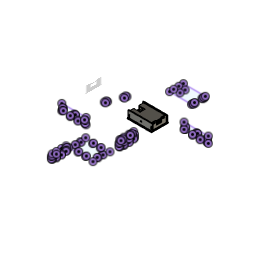
widgetlab1case (Autodesk Fusion 360 design; units mm, degrees)
Autodesk Fusion 360 part; units mm, degrees
(part 1 of 2)
sketch "base" plane through (0, 0, 0) normal (0, 0, 1) x (1, 0, 0)
  line L0 (-26.4, -40.65) -> (26.4, -40.65)
  line L1 (26.4, -40.65) -> (26.4, 40.65)
  line L2 (26.4, 40.65) -> (-26.4, 40.65)
  line L3 (-26.4, 40.65) -> (-26.4, -40.65)
  line L4 (-26.4, -40.65) -> (26.4, -40.65)
  dimension "d5" = 81.3
  dimension "d6" = 52.8
  dimension "d58" = 26.4
  dimension "d59" = 40.65
  dimension "d81" = 52.8
  constraint horizontal L0
  constraint vertical L1
  constraint horizontal L2
  constraint vertical L3
  constraint horizontal L4
  measures "d5" distance of L0.start L2.end
  measures "d6" distance of L1.end L2.end
  measures "d58" distance of origin L1
  measures "d59" distance of origin L2
  measures "d81" distance of L0.start L0.end
extrude "Extrude1" add sketch "base" along normal blind 9.7 makes body 1
sketch "centre groove" plane through (0, 0, 9.7) normal (0, 0, 1) x (1, 0, 0)
  line L0 (-26.4, 40.65) -> (-26.4, -40.65)
  line L1 (-26.4, -40.65) -> (26.4, -40.65)
  line L2 (26.4, -40.65) -> (26.4, 40.65)
  line L3 (26.4, 40.65) -> (-26.4, 40.65)
  line L4 (1.1, -40.65) -> (-1.1, -40.65)
  line L5 (-1.1, -40.65) -> (-1.1, 40.65)
  line L6 (-1.1, 40.65) -> (1.1, 40.65)
  line L7 (1.1, 40.65) -> (1.1, -40.65)
  line L8 (1.1, -40.65) -> (-1.1, 40.65) construction
  line L9 (-1.1, -40.65) -> (1.1, 40.65) construction
  line L10 (-1.1, -40.65) -> (0, -40.65)
  dimension "d9" = 2.2
  dimension "d11" = 1.1
  dimension "d60" = 40.65
  constraint horizontal L4
  constraint perpendicular L4 L5
  constraint parallel L4 L6
  constraint parallel L5 L7
  constraint coincident L8 origin
  constraint coincident L9 origin
  constraint perpendicular L5 L10
  measures "d9" distance of L5.end L6.end
  measures "d11" distance of L4.end L10.end
  measures "d60" distance of L6 origin
extrude "Extrude2" cut sketch "centre groove" against normal blind 3 contours L1 L3 L4 L5 L6 L7 L10 bodies 1
sketch "side dots" plane through (0, 0, 0) normal (0, 0, 1) x (1, 0, 0)
  line L0 (-26.4, 40.65) -> (-26.4, -40.65) construction
  line L1 (26.4, -40.65) -> (26.4, 40.65) construction
  line L2 (26.4, 40.65) -> (1.1, 40.65) construction
  line L3 (-1.1, 40.65) -> (-26.4, 40.65) construction
  line L4 (-1.1, 40.65) -> (1.1, 40.65) construction
  line L5 (-26.4, -40.65) -> (-1.1, -40.65) construction
  line L6 (1.1, -40.65) -> (-1.1, -40.65) construction
  line L7 (1.1, -40.65) -> (26.4, -40.65) construction
  line L8 (-26.4, -40.65) -> (-26.4, -27.3)
  line L9 (-26.4, -27.3) -> (-26.4, 27.3)
  line L10 (0, -40.65) -> (22.3, -40.65)
  line L11 (0, -40.65) -> (-22.3, -40.65)
  line L12 (-26.4, 27.3) -> (-27, 27.3)
  line L13 (-26.4, -27.3) -> (-27, -27.3)
  line L14 (-22.3, -40.65) -> (-22.3, -41.25)
  line L15 (22.3, -40.65) -> (22.3, -41.25)
  circle A0 centre (-27, 27.3) radius 1
  circle A1 centre (-27, -27.3) radius 1
  circle A2 centre (-22.3, -41.25) radius 1
  circle A3 centre (22.3, -41.25) radius 1
  circle A4 centre (0, -41.25) radius 1
  line L16 (0, -40.65) -> (0, -41.25)
  point P0 (-1.1, 40.65)
  point P1 (-1.1, 40.65)
  dimension "d14" = 13.35
  dimension "d15" = 54.6
  dimension "d16" = 22.3
  dimension "d17" = 22.3
  dimension "d18" = 0.6
  dimension "d19" = 0.6
  dimension "d20" = 0.6
  dimension "d21" = 0.6
  dimension "d22" = 2
  dimension "d23" = 2
  dimension "d24" = 2
  dimension "d25" = 2
  dimension "d26" = 2
  dimension "d27" = 0.6
  constraint coincident L0.end L5.start
  constraint perpendicular L5 L8
  constraint parallel L0 L9
  constraint midpoint L6 L10.start
  constraint perpendicular L1 L10
  constraint parallel L5 L11
  constraint perpendicular L9 L12
  constraint perpendicular L0 L13
  constraint perpendicular L11 L14
  constraint perpendicular L10 L15
  constraint coincident L12.end A0.centre
  constraint coincident L13.end A1.centre
  constraint coincident L14.end A2.centre
  constraint coincident L15.end A3.centre
  constraint perpendicular L11 L16
  constraint coincident A4.centre L16.end
  measures "d14" distance of L0.end L8.end
  measures "d15" distance of L8.end L9.end
  measures "d16" distance of L10.start L10.end
  measures "d17" distance of L10.start L11.end
  measures "d18" distance of L9.end L12.end
  measures "d19" distance of L8.end L13.end
  measures "d20" distance of L11.end L14.end
  measures "d21" distance of L10.end L15.end
  measures "d22" diameter of A0
  measures "d23" diameter of A1
  measures "d24" diameter of A2
  measures "d25" diameter of A3
  measures "d26" diameter of A4
  measures "d27" distance of L10.start A4.centre
extrude "Extrude3" add sketch "side dots" along normal blind 4.8 contours L8 L9 A1 | L10 L11 A4 | A0 | A2 | A3 picked at (-27.463, -27.251) picked at (0.0281, -41.7143) bodies 1
sketch "holes" plane through (0, 0, 9.7) normal (0, 0, 1) x (1, 0, 0)
  line L0 (-1.1, -40.65) -> (-1.1, 40.65)
  line L1 (-1.1, 40.65) -> (-26.4, 40.65)
  line L2 (-26.4, 40.65) -> (-26.4, -40.65)
  line L3 (-26.4, -40.65) -> (-1.1, -40.65)
  line L4 (20, 0) -> (2.5, 0)
  line L5 (0, 2.5) -> (0, 20)
  line L6 (0, 0) -> (-26.4, 0) construction
  point P0 (-3.8, 1.27)
  point P1 (-6.34, 1.27)
  point P2 (-8.88, 1.27)
  point P3 (-11.42, 1.27)
  point P4 (-13.96, 1.27)
  point P5 (-3.8, 3.81)
  point P6 (-6.34, 3.81)
  point P7 (-8.88, 3.81)
  point P8 (-11.42, 3.81)
  point P9 (-13.96, 3.81)
  point P10 (-3.8, 6.35)
  point P11 (-6.34, 6.35)
  point P12 (-8.88, 6.35)
  point P13 (-11.42, 6.35)
  point P14 (-13.96, 6.35)
  point P15 (-3.8, 8.89)
  point P16 (-6.34, 8.89)
  point P17 (-8.88, 8.89)
  point P18 (-11.42, 8.89)
  point P19 (-13.96, 8.89)
  point P20 (-3.8, 11.43)
  point P21 (-6.34, 11.43)
  point P22 (-8.88, 11.43)
  point P23 (-11.42, 11.43)
  point P24 (-13.96, 11.43)
  point P25 (-3.8, 13.97)
  point P26 (-6.34, 13.97)
  point P27 (-8.88, 13.97)
  point P28 (-11.42, 13.97)
  point P29 (-13.96, 13.97)
  point P30 (-3.8, 16.51)
  point P31 (-6.34, 16.51)
  point P32 (-8.88, 16.51)
  point P33 (-11.42, 16.51)
  point P34 (-13.96, 16.51)
  point P35 (-3.8, 19.05)
  point P36 (-6.34, 19.05)
  point P37 (-8.88, 19.05)
  point P38 (-11.42, 19.05)
  point P39 (-13.96, 19.05)
  point P40 (-3.8, 21.59)
  point P41 (-6.34, 21.59)
  point P42 (-8.88, 21.59)
  point P43 (-11.42, 21.59)
  point P44 (-13.96, 21.59)
  point P45 (-3.8, 24.13)
  point P46 (-6.34, 24.13)
  point P47 (-8.88, 24.13)
  point P48 (-11.42, 24.13)
  point P49 (-13.96, 24.13)
  point P50 (-3.8, 26.67)
  point P51 (-6.34, 26.67)
  point P52 (-8.88, 26.67)
  point P53 (-11.42, 26.67)
  point P54 (-13.96, 26.67)
  point P55 (-3.8, 29.21)
  point P56 (-6.34, 29.21)
  point P57 (-8.88, 29.21)
  point P58 (-11.42, 29.21)
  point P59 (-13.96, 29.21)
  point P60 (-3.8, 31.75)
  point P61 (-6.34, 31.75)
  point P62 (-8.88, 31.75)
  point P63 (-11.42, 31.75)
  point P64 (-13.96, 31.75)
  point P65 (-3.8, 34.29)
  point P66 (-6.34, 34.29)
  point P67 (-8.88, 34.29)
  point P68 (-11.42, 34.29)
  point P69 (-13.96, 34.29)
  point P70 (-3.8, 36.83)
  point P71 (-6.34, 36.83)
  point P72 (-8.88, 36.83)
  point P73 (-11.42, 36.83)
  point P74 (-13.96, 36.83)
  point P75 (-20.71, 0)
  point P76 (-20.71, -5.08)
  point P77 (-23.25, -5.08)
  point P78 (-20.71, -2.54)
  point P79 (-23.25, -2.54)
  point P80 (-23.25, 0)
  point P81 (-20.71, 2.54)
  point P82 (-23.25, 2.54)
  point P83 (-20.71, 5.08)
  point P84 (-23.25, 5.08)
  point P85 (-23.25, -25.4)
  point P86 (-20.71, -25.4)
  point P87 (-23.25, -27.94)
  point P88 (-20.71, -27.94)
  point P89 (-23.25, -30.48)
  point P90 (-20.71, -30.48)
  point P91 (-23.25, -33.02)
  point P92 (-20.71, -33.02)
  point P93 (-23.25, -35.56)
  point P94 (-20.71, -35.56)
  point P95 (-23.25, -10.16)
  point P96 (-20.71, -10.16)
  point P97 (-23.25, -12.7)
  point P98 (-20.71, -12.7)
  point P99 (-23.25, -15.24)
  point P100 (-20.71, -15.24)
  point P101 (-23.25, -17.78)
  point P102 (-20.71, -17.78)
  point P103 (-23.25, -20.32)
  point P104 (-20.71, -20.32)
  point P105 (-23.25, 20.32)
  point P106 (-20.71, 20.32)
  point P107 (-23.25, 17.78)
  point P108 (-20.71, 17.78)
  point P109 (-23.25, 15.24)
  point P110 (-20.71, 15.24)
  point P111 (-23.25, 12.7)
  point P112 (-20.71, 12.7)
  point P113 (-23.25, 10.16)
  point P114 (-20.71, 10.16)
  point P115 (-23.25, 35.56)
  point P116 (-20.71, 35.56)
  point P117 (-23.25, 33.02)
  point P118 (-20.71, 33.02)
  point P119 (-23.25, 30.48)
  point P120 (-20.71, 30.48)
  point P121 (-23.25, 27.94)
  point P122 (-20.71, 27.94)
  point P123 (-23.25, 25.4)
  point P124 (-20.71, 25.4)
  point P125 (-13.96, -31.75)
  point P126 (-13.96, -34.29)
  point P127 (-13.96, -36.83)
  point P128 (-3.8, -31.75)
  point P129 (-11.42, -31.75)
  point P130 (-3.8, -24.13)
  point P131 (-3.8, -36.83)
  point P132 (-6.34, -21.59)
  point P133 (-3.8, -29.21)
  point P134 (-8.88, -29.21)
  point P135 (-6.34, -36.83)
  point P136 (-8.88, -31.75)
  point P137 (-13.96, -21.59)
  point P138 (-13.96, -3.81)
  point P139 (-8.88, -21.59)
  point P140 (-3.8, -34.29)
  point P141 (-8.88, -34.29)
  point P142 (-11.42, -36.83)
  point P143 (-11.42, -8.89)
  point P144 (-8.88, -11.43)
  point P145 (-8.88, -36.83)
  point P146 (-13.96, -6.35)
  point P147 (-13.96, -11.43)
  point P148 (-6.34, -24.13)
  point P149 (-6.34, -29.21)
  point P150 (-13.96, -1.27)
  point P151 (-8.88, -26.67)
  point P152 (-3.8, -21.59)
  point P153 (-11.42, -34.29)
  point P154 (-6.34, -26.67)
  point P155 (-11.42, -13.97)
  point P156 (-6.34, -31.75)
  point P157 (-13.96, -16.51)
  point P158 (-11.42, -11.43)
  point P159 (-11.42, -26.67)
  point P160 (-6.34, -19.05)
  point P161 (-8.88, -19.05)
  point P162 (-13.96, -8.89)
  point P163 (-11.42, -19.05)
  point P164 (-11.42, -24.13)
  point P165 (-11.42, -21.59)
  point P166 (-13.96, -26.67)
  point P167 (-13.96, -29.21)
  point P168 (-3.8, -26.67)
  point P169 (-11.42, -1.27)
  point P170 (-8.88, -8.89)
  point P171 (-11.42, -29.21)
  point P172 (-11.42, -6.35)
  point P173 (-6.34, -34.29)
  point P174 (-13.96, -24.13)
  point P175 (-13.96, -13.97)
  point P176 (-8.88, -1.27)
  point P177 (-3.8, -8.89)
  point P178 (-3.8, -6.35)
  point P179 (-8.88, -6.35)
  point P180 (-11.42, -3.81)
  point P181 (-8.88, -16.51)
  point P182 (-6.34, -1.27)
  point P183 (-11.42, -16.51)
  point P184 (-3.8, -3.81)
  point P185 (-6.34, -8.89)
  point P186 (-6.34, -6.35)
  point P187 (-3.8, -11.43)
  point P188 (-6.34, -11.43)
  point P189 (-6.34, -16.51)
  point P190 (-8.88, -3.81)
  point P191 (-8.88, -24.13)
  point P192 (-6.34, -13.97)
  point P193 (-8.88, -13.97)
  point P194 (-3.8, -19.05)
  point P195 (-3.8, -16.51)
  point P196 (-3.8, -13.97)
  point P197 (-6.34, -3.81)
  point P198 (-13.96, -19.05)
  point P199 (-3.8, -1.27)
  point P200 (3.8, -21.59)
  point P201 (8.88, 34.29)
  point P202 (13.96, 1.27)
  point P203 (20.71, -15.24)
  point P204 (23.25, 5.08)
  point P205 (6.34, 13.97)
  point P206 (11.42, -36.83)
  point P207 (3.8, -6.35)
  point P208 (3.8, 1.27)
  point P209 (23.25, -27.94)
  point P210 (3.8, 36.83)
  point P211 (11.42, -29.21)
  point P212 (6.34, 3.81)
  point P213 (11.42, -8.89)
  point P214 (13.96, -13.97)
  point P215 (23.25, 17.78)
  point P216 (8.88, 29.21)
  point P217 (20.71, 10.16)
  point P218 (13.96, 36.83)
  point P219 (3.8, -26.67)
  point P220 (8.88, -24.13)
  point P221 (23.25, -17.78)
  point P222 (13.96, -31.75)
  point P223 (8.88, 8.89)
  point P224 (3.8, 31.75)
  point P225 (8.88, 31.75)
  point P226 (20.71, -12.7)
  point P227 (6.34, -16.51)
  point P228 (11.42, -13.97)
  point P229 (11.42, -16.51)
  point P230 (3.8, -3.81)
  point P231 (20.71, 17.78)
  point P232 (6.34, -11.43)
  point P233 (3.8, 24.13)
  point P234 (13.96, -34.29)
  point P235 (23.25, -20.32)
  point P236 (20.71, -30.48)
  point P237 (6.34, 29.21)
  point P238 (20.71, 33.02)
  point P239 (6.34, 11.43)
  point P240 (8.88, 16.51)
  point P241 (13.96, 26.67)
  point P242 (11.42, 6.35)
  point P243 (8.88, -8.89)
  point P244 (11.42, -11.43)
  point P245 (13.96, -21.59)
  point P246 (13.96, 34.29)
  point P247 (3.8, -31.75)
  point P248 (11.42, -31.75)
  point P249 (6.34, -21.59)
  point P250 (11.42, 1.27)
  point P251 (20.71, -20.32)
  point P252 (8.88, -26.67)
  point P253 (6.34, -34.29)
  point P254 (3.8, 8.89)
  point P255 (13.96, -19.05)
  point P256 (23.25, -25.4)
  point P257 (6.34, -29.21)
  point P258 (23.25, -33.02)
  point P259 (3.8, 34.29)
  point P260 (8.88, -11.43)
  point P261 (23.25, 35.56)
  point P262 (3.8, -1.27)
  point P263 (13.96, 29.21)
  point P264 (3.8, 29.21)
  point P265 (3.8, -34.29)
  point P266 (8.88, -29.21)
  point P267 (23.25, 33.02)
  point P268 (13.96, -24.13)
  point P269 (11.42, 36.83)
  point P270 (8.88, -13.97)
  point P271 (8.88, -31.75)
  point P272 (13.96, -26.67)
  point P273 (6.34, -26.67)
  point P274 (3.8, 19.05)
  point P275 (3.8, 6.35)
  point P276 (11.42, -24.13)
  point P277 (20.71, -27.94)
  point P278 (8.88, 24.13)
  point P279 (6.34, 1.27)
  point P280 (6.34, -36.83)
  point P281 (11.42, 34.29)
  point P282 (8.88, 3.81)
  point P283 (23.25, -30.48)
  point P284 (11.42, -34.29)
  point P285 (3.8, -8.89)
  point P286 (6.34, -1.27)
  point P287 (8.88, -3.81)
  point P288 (3.8, 16.51)
  point P289 (11.42, 29.21)
  point P290 (8.88, 11.43)
  point P291 (23.25, 30.48)
  point P292 (3.8, -11.43)
  point P293 (20.71, -35.56)
  point P294 (13.96, -16.51)
  point P295 (23.25, -35.56)
  point P296 (3.8, -24.13)
  point P297 (13.96, -11.43)
  point P298 (3.8, 11.43)
  point P299 (20.71, 35.56)
  point P300 (13.96, -36.83)
  point P301 (6.34, -6.35)
  point P302 (3.8, -36.83)
  point P303 (11.42, 31.75)
  point P304 (6.34, -8.89)
  point P305 (3.8, -16.51)
  point P306 (13.96, 21.59)
  point P307 (11.42, -26.67)
  point P308 (6.34, -31.75)
  point P309 (8.88, -1.27)
  point P310 (8.88, 36.83)
  point P311 (11.42, -21.59)
  point P312 (20.71, -25.4)
  point P313 (11.42, -6.35)
  point P314 (20.71, 5.08)
  point P315 (11.42, 21.59)
  point P316 (13.96, 16.51)
  point P317 (13.96, 6.35)
  point P318 (11.42, 11.43)
  point P319 (8.88, 19.05)
  point P320 (6.34, 24.13)
  point P321 (13.96, -1.27)
  point P322 (23.25, 2.54)
  point P323 (23.25, -2.54)
  point P324 (11.42, 16.51)
  point P325 (11.42, 8.89)
  point P326 (13.96, 3.81)
  point P327 (13.96, 19.05)
  point P328 (20.71, -2.54)
  point P329 (13.96, 11.43)
  point P330 (13.96, -3.81)
  point P331 (23.25, 10.16)
  point P332 (20.71, 15.24)
  point P333 (23.25, 0)
  point P334 (13.96, 13.97)
  point P335 (11.42, -3.81)
  point P336 (11.42, -1.27)
  point P337 (11.42, 19.05)
  point P338 (20.71, -17.78)
  point P339 (23.25, 20.32)
  point P340 (23.25, 15.24)
  point P341 (8.88, 26.67)
  point P342 (6.34, 19.05)
  point P343 (6.34, 21.59)
  point P344 (20.71, 25.4)
  point P345 (13.96, 8.89)
  point P346 (20.71, -10.16)
  point P347 (23.25, -5.08)
  point P348 (11.42, 26.67)
  point P349 (20.71, 2.54)
  point P350 (6.34, 26.67)
  point P351 (20.71, 20.32)
  point P352 (11.42, -19.05)
  point P353 (11.42, 13.97)
  point P354 (23.25, -12.7)
  point P355 (13.96, 24.13)
  point P356 (8.88, 21.59)
  point P357 (20.71, 0)
  point P358 (13.96, -6.35)
  point P359 (20.71, 12.7)
  point P360 (23.25, 25.4)
  point P361 (20.71, -5.08)
  point P362 (23.25, 12.7)
  point P363 (3.8, 21.59)
  point P364 (11.42, 3.81)
  point P365 (3.8, 26.67)
  point P366 (8.88, -16.51)
  point P367 (3.8, 13.97)
  point P368 (6.34, 16.51)
  point P369 (23.25, -15.24)
  point P370 (6.34, 31.75)
  point P371 (6.34, 34.29)
  point P372 (13.96, -29.21)
  point P373 (6.34, -19.05)
  point P374 (20.71, -33.02)
  point P375 (3.8, -19.05)
  point P376 (8.88, 6.35)
  point P377 (13.96, 31.75)
  point P378 (20.71, 30.48)
  point P379 (8.88, -6.35)
  point P380 (3.8, 3.81)
  point P381 (8.88, -34.29)
  point P382 (8.88, 1.27)
  point P383 (6.34, -3.81)
  point P384 (6.34, -13.97)
  point P385 (8.88, -19.05)
  point P386 (8.88, 13.97)
  point P387 (6.34, 6.35)
  point P388 (20.71, 27.94)
  point P389 (23.25, -10.16)
  point P390 (23.25, 27.94)
  point P391 (6.34, -24.13)
  point P392 (8.88, -21.59)
  point P393 (13.96, -8.89)
  point P394 (11.42, 24.13)
  point P395 (8.88, -36.83)
  point P396 (6.34, 36.83)
  point P397 (6.34, 8.89)
  point P398 (3.8, -13.97)
  point P399 (3.8, -29.21)
  dimension "d32" = 3.8
  dimension "d33" = 1.27
  dimension "d36" = -10.16
  dimension "d37" = 35.56
  dimension "d39" = 6.75
  dimension "d42" = -2.54
  dimension "d43" = 5.08
  dimension "d46" = 0
  dimension "d47" = 30.48
  constraint symmetric P0 L4 P199
  constraint symmetric P1 L4 P182
  constraint symmetric P2 L4 P176
  constraint symmetric P3 L4 P169
  constraint symmetric P4 L4 P150
  constraint symmetric P5 L4 P184
  constraint symmetric P6 L4 P197
  constraint symmetric P7 L4 P190
  constraint symmetric P8 L4 P180
  constraint symmetric P9 L4 P138
  constraint symmetric P10 L4 P178
  constraint symmetric P11 L4 P186
  constraint symmetric P12 L4 P179
  constraint symmetric P13 L4 P172
  constraint symmetric P14 L4 P146
  constraint symmetric P15 L4 P177
  constraint symmetric P16 L4 P185
  constraint symmetric P17 L4 P170
  constraint symmetric P18 L4 P143
  constraint symmetric P19 L4 P162
  constraint symmetric P20 L4 P187
  constraint symmetric P21 L4 P188
  constraint symmetric P22 L4 P144
  constraint symmetric P23 L4 P158
  constraint symmetric P24 L4 P147
  constraint symmetric P25 L4 P196
  constraint symmetric P26 L4 P192
  constraint symmetric P27 L4 P193
  constraint symmetric P28 L4 P155
  constraint symmetric P29 L4 P175
  constraint symmetric P30 L4 P195
  constraint symmetric P31 L4 P189
  constraint symmetric P32 L4 P181
  constraint symmetric P33 L4 P183
  constraint symmetric P34 L4 P157
  constraint symmetric P35 L4 P194
  constraint symmetric P36 L4 P160
  constraint symmetric P37 L4 P161
  constraint symmetric P38 L4 P163
  constraint symmetric P39 L4 P198
  constraint symmetric P40 L4 P152
  constraint symmetric P41 L4 P132
  constraint symmetric P42 L4 P139
  constraint symmetric P43 L4 P165
  constraint symmetric P44 L4 P137
  constraint symmetric P45 L4 P130
  constraint symmetric P46 L4 P148
  constraint symmetric P47 L4 P191
  constraint symmetric P48 L4 P164
  constraint symmetric P49 L4 P174
  constraint symmetric P50 L4 P168
  constraint symmetric P51 L4 P154
  constraint symmetric P52 L4 P151
  constraint symmetric P53 L4 P159
  constraint symmetric P54 L4 P166
  constraint symmetric P55 L4 P133
  constraint symmetric P56 L4 P149
  constraint symmetric P57 L4 P134
  constraint symmetric P58 L4 P171
  constraint symmetric P59 L4 P167
  constraint symmetric P60 L4 P128
  constraint symmetric P61 L4 P156
  constraint symmetric P62 L4 P136
  constraint symmetric P63 L4 P129
  constraint symmetric P64 L4 P125
  constraint symmetric P65 L4 P140
  constraint symmetric P66 L4 P173
  constraint symmetric P67 L4 P141
  constraint symmetric P68 L4 P153
  constraint symmetric P69 L4 P126
  constraint symmetric P70 L4 P131
  constraint symmetric P71 L4 P135
  constraint symmetric P72 L4 P145
  constraint symmetric P73 L4 P142
  constraint symmetric P74 L4 P127
  constraint symmetric P0 L5 P208
  constraint symmetric P1 L5 P279
  constraint symmetric P2 L5 P382
  constraint symmetric P3 L5 P250
  constraint symmetric P4 L5 P202
  constraint symmetric P5 L5 P380
  constraint symmetric P6 L5 P212
  constraint symmetric P7 L5 P282
  constraint symmetric P8 L5 P364
  constraint symmetric P9 L5 P326
  constraint symmetric P10 L5 P275
  constraint symmetric P11 L5 P387
  constraint symmetric P12 L5 P376
  constraint symmetric P13 L5 P242
  constraint symmetric P14 L5 P317
  constraint symmetric P15 L5 P254
  constraint symmetric P16 L5 P397
  constraint symmetric P17 L5 P223
  constraint symmetric P18 L5 P325
  constraint symmetric P19 L5 P345
  constraint symmetric P20 L5 P298
  constraint symmetric P21 L5 P239
  constraint symmetric P22 L5 P290
  constraint symmetric P23 L5 P318
  constraint symmetric P24 L5 P329
  constraint symmetric P25 L5 P367
  constraint symmetric P26 L5 P205
  constraint symmetric P27 L5 P386
  constraint symmetric P28 L5 P353
  constraint symmetric P29 L5 P334
  constraint symmetric P30 L5 P288
  constraint symmetric P31 L5 P368
  constraint symmetric P32 L5 P240
  constraint symmetric P33 L5 P324
  constraint symmetric P34 L5 P316
  constraint symmetric P35 L5 P274
  constraint symmetric P36 L5 P342
  constraint symmetric P37 L5 P319
  constraint symmetric P38 L5 P337
  constraint symmetric P39 L5 P327
  constraint symmetric P40 L5 P363
  constraint symmetric P41 L5 P343
  constraint symmetric P42 L5 P356
  constraint symmetric P43 L5 P315
  constraint symmetric P44 L5 P306
  constraint symmetric P45 L5 P233
  constraint symmetric P46 L5 P320
  constraint symmetric P47 L5 P278
  constraint symmetric P48 L5 P394
  constraint symmetric P49 L5 P355
  constraint symmetric P50 L5 P365
  constraint symmetric P51 L5 P350
  constraint symmetric P52 L5 P341
  constraint symmetric P53 L5 P348
  constraint symmetric P54 L5 P241
  constraint symmetric P55 L5 P264
  constraint symmetric P56 L5 P237
  constraint symmetric P57 L5 P216
  constraint symmetric P58 L5 P289
  constraint symmetric P59 L5 P263
  constraint symmetric P60 L5 P224
  constraint symmetric P61 L5 P370
  constraint symmetric P62 L5 P225
  constraint symmetric P63 L5 P303
  constraint symmetric P64 L5 P377
  constraint symmetric P65 L5 P259
  constraint symmetric P66 L5 P371
  constraint symmetric P67 L5 P201
  constraint symmetric P68 L5 P281
  constraint symmetric P69 L5 P246
  constraint symmetric P70 L5 P210
  constraint symmetric P71 L5 P396
  constraint symmetric P72 L5 P310
  constraint symmetric P73 L5 P269
  constraint symmetric P74 L5 P218
  constraint symmetric P75 L5 P357
  constraint symmetric P76 L5 P361
  constraint symmetric P77 L5 P347
  constraint symmetric P78 L5 P328
  constraint symmetric P79 L5 P323
  constraint symmetric P80 L5 P333
  constraint symmetric P81 L5 P349
  constraint symmetric P82 L5 P322
  constraint symmetric P83 L5 P314
  constraint symmetric P84 L5 P204
  constraint symmetric P85 L5 P256
  constraint symmetric P86 L5 P312
  constraint symmetric P87 L5 P209
  constraint symmetric P88 L5 P277
  constraint symmetric P89 L5 P283
  constraint symmetric P90 L5 P236
  constraint symmetric P91 L5 P258
  constraint symmetric P92 L5 P374
  constraint symmetric P93 L5 P295
  constraint symmetric P94 L5 P293
  constraint symmetric P95 L5 P389
  constraint symmetric P96 L5 P346
  constraint symmetric P97 L5 P354
  constraint symmetric P98 L5 P226
  constraint symmetric P99 L5 P369
  constraint symmetric P100 L5 P203
  constraint symmetric P101 L5 P221
  constraint symmetric P102 L5 P338
  constraint symmetric P103 L5 P235
  constraint symmetric P104 L5 P251
  constraint symmetric P105 L5 P339
  constraint symmetric P106 L5 P351
  constraint symmetric P107 L5 P215
  constraint symmetric P108 L5 P231
  constraint symmetric P109 L5 P340
  constraint symmetric P110 L5 P332
  constraint symmetric P111 L5 P362
  constraint symmetric P112 L5 P359
  constraint symmetric P113 L5 P331
  constraint symmetric P114 L5 P217
  constraint symmetric P115 L5 P261
  constraint symmetric P116 L5 P299
  constraint symmetric P117 L5 P267
  constraint symmetric P118 L5 P238
  constraint symmetric P119 L5 P291
  constraint symmetric P120 L5 P378
  constraint symmetric P121 L5 P390
  constraint symmetric P122 L5 P388
  constraint symmetric P123 L5 P360
  constraint symmetric P124 L5 P344
  constraint symmetric P125 L5 P222
  constraint symmetric P126 L5 P234
  constraint symmetric P127 L5 P300
  constraint symmetric P128 L5 P247
  constraint symmetric P129 L5 P248
  constraint symmetric P130 L5 P296
  constraint symmetric P131 L5 P302
  constraint symmetric P132 L5 P249
  constraint symmetric P133 L5 P399
  constraint symmetric P134 L5 P266
  constraint symmetric P135 L5 P280
  constraint symmetric P136 L5 P271
  constraint symmetric P137 L5 P245
  constraint symmetric P138 L5 P330
  constraint symmetric P139 L5 P392
  constraint symmetric P140 L5 P265
  constraint symmetric P141 L5 P381
  constraint symmetric P142 L5 P206
  constraint symmetric P143 L5 P213
  constraint symmetric P144 L5 P260
  constraint symmetric P145 L5 P395
  constraint symmetric P146 L5 P358
  constraint symmetric P147 L5 P297
  constraint symmetric P148 L5 P391
  constraint symmetric P149 L5 P257
  constraint symmetric P150 L5 P321
  constraint symmetric P151 L5 P252
  constraint symmetric P152 L5 P200
  constraint symmetric P153 L5 P284
  constraint symmetric P154 L5 P273
  constraint symmetric P155 L5 P228
  constraint symmetric P156 L5 P308
  constraint symmetric P157 L5 P294
  constraint symmetric P158 L5 P244
  constraint symmetric P159 L5 P307
  constraint symmetric P160 L5 P373
  constraint symmetric P161 L5 P385
  constraint symmetric P162 L5 P393
  constraint symmetric P163 L5 P352
  constraint symmetric P164 L5 P276
  constraint symmetric P165 L5 P311
  constraint symmetric P166 L5 P272
  constraint symmetric P167 L5 P372
  constraint symmetric P168 L5 P219
  constraint symmetric P169 L5 P336
  constraint symmetric P170 L5 P243
  constraint symmetric P171 L5 P211
  constraint symmetric P172 L5 P313
  constraint symmetric P173 L5 P253
  constraint symmetric P174 L5 P268
  constraint symmetric P175 L5 P214
  constraint symmetric P176 L5 P309
  constraint symmetric P177 L5 P285
  constraint symmetric P178 L5 P207
  constraint symmetric P179 L5 P379
  constraint symmetric P180 L5 P335
  constraint symmetric P181 L5 P366
  constraint symmetric P182 L5 P286
  constraint symmetric P183 L5 P229
  constraint symmetric P184 L5 P230
  constraint symmetric P185 L5 P304
  constraint symmetric P186 L5 P301
  constraint symmetric P187 L5 P292
  constraint symmetric P188 L5 P232
  constraint symmetric P189 L5 P227
  constraint symmetric P190 L5 P287
  constraint symmetric P191 L5 P220
  constraint symmetric P192 L5 P384
  constraint symmetric P193 L5 P270
  constraint symmetric P194 L5 P375
  constraint symmetric P195 L5 P305
  constraint symmetric P196 L5 P398
  constraint symmetric P197 L5 P383
  constraint symmetric P198 L5 P255
  constraint symmetric P199 L5 P262
  constraint coincident L6.start origin
  constraint midpoint L2 L6.end
  constraint coincident P80 L6
  measures "d24" diameter of P81
  measures "d25" diameter of P313
  measures "d32" horizontal distance of L6.start P0
  measures "d33" vertical distance of L6.start P0
  measures "d39" horizontal distance of P4 P75
hole "Hole1" at (-6.34, -1.27, 9.7) at (-20.71, -10.16, 9.7) at (-3.8, 13.97, 9.7) at (-13.96, 8.89, 9.7) at (-6.34, -13.97, 9.7) at (-8.88, -24.13, 9.7) at (-3.8, -3.81, 9.7) at (-13.96, 34.29, 9.7) at (-23.25, -35.56, 9.7) at (-20.71, -33.02, 9.7) at (-20.71, -12.7, 9.7) at (-3.8, 11.43, 9.7) at (-20.71, 20.32, 9.7) at (-8.88, -1.27, 9.7) at (-13.96, 13.97, 9.7) at (-11.42, 13.97, 9.7) at (-8.88, 36.83, 9.7) at (-3.8, -36.83, 9.7) at (-8.88, 11.43, 9.7) at (-20.71, -30.48, 9.7) at (-13.96, 29.21, 9.7) at (-13.96, -13.97, 9.7) at (-3.8, -21.59, 9.7) at (-13.96, -1.27, 9.7) at (-6.34, -16.51, 9.7) at (-3.8, 3.81, 9.7) at (-11.42, 19.05, 9.7) at (-23.25, -17.78, 9.7) at (-3.8, -31.75, 9.7) at (-11.42, -24.13, 9.7) at (-8.88, 6.35, 9.7) at (-6.34, -6.35, 9.7) at (-3.8, 34.29, 9.7) at (-13.96, -11.43, 9.7) at (-13.96, 19.05, 9.7) at (-8.88, -11.43, 9.7) at (-3.8, -24.13, 9.7) at (-8.88, -3.81, 9.7) at (-13.96, -21.59, 9.7) at (-13.96, 36.83, 9.7) at (-6.34, 8.89, 9.7) at (-8.88, -13.97, 9.7) at (-20.71, -35.56, 9.7) at (-3.8, 16.51, 9.7) at (-8.88, 29.21, 9.7) at (-6.34, -31.75, 9.7) at (-20.71, 12.7, 9.7) at (-23.25, -25.4, 9.7) at (-6.34, -24.13, 9.7) at (-20.71, -20.32, 9.7) at (-23.25, 20.32, 9.7) at (-8.88, -16.51, 9.7) at (-11.42, -36.83, 9.7) at (-6.34, -36.83, 9.7) at (-3.8, -19.05, 9.7) at (-3.8, 19.05, 9.7) at (-8.88, -6.35, 9.7) at (-20.71, -25.4, 9.7) at (-6.34, 29.21, 9.7) at (-11.42, -16.51, 9.7) at (-3.8, 1.27, 9.7) at (-6.34, -21.59, 9.7) at (-6.34, -11.43, 9.7) at (-8.88, -31.75, 9.7) at (-6.34, 6.35, 9.7) at (-6.34, 24.13, 9.7) at (-13.96, -29.21, 9.7) at (-8.88, 26.67, 9.7) at (-13.96, 31.75, 9.7) at (-13.96, 21.59, 9.7) at (-20.71, 10.16, 9.7) at (-3.8, 29.21, 9.7) at (-11.42, 26.67, 9.7) at (-20.71, -27.94, 9.7) at (-6.34, -26.67, 9.7) at (-3.8, 26.67, 9.7) at (-3.8, 6.35, 9.7) at (-8.88, 3.81, 9.7) at (-8.88, -34.29, 9.7) at (-23.25, -5.08, 9.7) at (-3.8, -1.27, 9.7) at (-13.96, -8.89, 9.7) at (-8.88, -21.59, 9.7) at (-11.42, -21.59, 9.7) at (-3.8, 24.13, 9.7) at (-11.42, 8.89, 9.7) at (-6.34, 3.81, 9.7) at (-8.88, 31.75, 9.7) at (-6.34, 31.75, 9.7) at (-20.71, 30.48, 9.7) at (-13.96, 26.67, 9.7) at (-13.96, 6.35, 9.7) at (-11.42, 16.51, 9.7) at (-23.25, 10.16, 9.7) at (-13.96, 16.51, 9.7) at (-11.42, 31.75, 9.7) at (-11.42, 29.21, 9.7) at (-23.25, 5.08, 9.7) at (-13.96, -19.05, 9.7) at (-11.42, -11.43, 9.7) at (-11.42, -26.67, 9.7) at (-20.71, -15.24, 9.7) at (-23.25, 27.94, 9.7) at (-6.34, 19.05, 9.7) at (-13.96, -3.81, 9.7) at (-23.25, 33.02, 9.7) at (-11.42, 21.59, 9.7) at (-11.42, -3.81, 9.7) at (-23.25, 35.56, 9.7) at (-6.34, 34.29, 9.7) at (-13.96, 1.27, 9.7) at (-13.96, 24.13, 9.7) at (-11.42, -6.35, 9.7) at (-13.96, 3.81, 9.7) at (-23.25, 2.54, 9.7) at (-13.96, 11.43, 9.7) at (-20.71, 2.54, 9.7) at (-13.96, -6.35, 9.7) at (-23.25, 15.24, 9.7) at (-11.42, 6.35, 9.7) at (-20.71, 15.24, 9.7) at (-11.42, 11.43, 9.7) at (-23.25, 0, 9.7) at (-20.71, 0, 9.7) at (-20.71, -5.08, 9.7) at (-11.42, -1.27, 9.7) at (-8.88, 16.51, 9.7) at (-20.71, 33.02, 9.7) at (-8.88, 21.59, 9.7) at (-23.25, -33.02, 9.7) at (-13.96, -24.13, 9.7) at (-20.71, -17.78, 9.7) at (-13.96, -34.29, 9.7) at (-11.42, 1.27, 9.7) at (-13.96, -31.75, 9.7) at (-23.25, 25.4, 9.7) at (-11.42, 36.83, 9.7) at (-8.88, -8.89, 9.7) at (-3.8, -26.67, 9.7) at (-3.8, -16.51, 9.7) at (-23.25, -20.32, 9.7) at (-3.8, -29.21, 9.7) at (-6.34, -34.29, 9.7) at (-20.71, 5.08, 9.7) at (-6.34, 1.27, 9.7) at (-11.42, 34.29, 9.7) at (-8.88, 24.13, 9.7) at (-3.8, 21.59, 9.7) at (-3.8, -6.35, 9.7) at (-11.42, -31.75, 9.7) at (-11.42, -13.97, 9.7) at (-11.42, 3.81, 9.7) at (-13.96, -16.51, 9.7) at (-13.96, -26.67, 9.7) at (-6.34, 16.51, 9.7) at (-6.34, 13.97, 9.7) at (-23.25, -2.54, 9.7) at (-3.8, 8.89, 9.7) at (-11.42, -29.21, 9.7) at (-8.88, 34.29, 9.7) at (-8.88, 1.27, 9.7) at (-23.25, -30.48, 9.7) at (-11.42, -19.05, 9.7) at (-20.71, 27.94, 9.7) at (-8.88, -36.83, 9.7) at (-3.8, 31.75, 9.7) at (-20.71, 35.56, 9.7) at (-6.34, -8.89, 9.7) at (-11.42, -34.29, 9.7) at (-20.71, -2.54, 9.7) at (-6.34, -3.81, 9.7) at (-8.88, -29.21, 9.7) at (-20.71, 25.4, 9.7) at (-6.34, 11.43, 9.7) at (-23.25, -12.7, 9.7) at (-6.34, 26.67, 9.7) at (-3.8, -13.97, 9.7) at (-6.34, -19.05, 9.7) at (-6.34, -29.21, 9.7) at (-3.8, -11.43, 9.7) at (-23.25, 30.48, 9.7) at (-23.25, -10.16, 9.7) at (-23.25, 12.7, 9.7) at (-20.71, 17.78, 9.7) at (-23.25, 17.78, 9.7) at (-11.42, -8.89, 9.7) at (-6.34, 21.59, 9.7) at (-8.88, 19.05, 9.7) at (-13.96, -36.83, 9.7) at (-11.42, 24.13, 9.7) at (-23.25, -15.24, 9.7) at (-23.25, -27.94, 9.7) at (-3.8, -34.29, 9.7) at (-3.8, 36.83, 9.7) at (-3.8, -8.89, 9.7) at (-8.88, -26.67, 9.7) at (-8.88, 8.89, 9.7) at (-8.88, -19.05, 9.7) at (-6.34, 36.83, 9.7) at (-8.88, 13.97, 9.7) direction (0, 0, -1) diameter 1.524 depth 7 tip angle 180 bodies 1
hole "Hole2" at (6.34, -11.43, 9.7) at (20.71, 15.24, 9.7) at (23.25, 2.54, 9.7) at (23.25, 0, 9.7) at (6.34, 34.29, 9.7) at (6.34, -26.67, 9.7) at (8.88, 11.43, 9.7) at (3.8, 1.27, 9.7) at (8.88, 26.67, 9.7) at (23.25, -17.78, 9.7) at (20.71, -33.02, 9.7) at (6.34, 13.97, 9.7) at (3.8, -8.89, 9.7) at (8.88, -26.67, 9.7) at (23.25, 17.78, 9.7) at (20.71, 17.78, 9.7) at (8.88, -29.21, 9.7) at (13.96, -21.59, 9.7) at (3.8, -29.21, 9.7) at (3.8, 16.51, 9.7) at (8.88, -31.75, 9.7) at (3.8, 26.67, 9.7) at (3.8, -16.51, 9.7) at (6.34, 8.89, 9.7) at (6.34, -6.35, 9.7) at (11.42, 1.27, 9.7) at (23.25, 25.4, 9.7) at (8.88, -1.27, 9.7) at (13.96, 6.35, 9.7) at (8.88, 3.81, 9.7) at (6.34, -16.51, 9.7) at (13.96, -3.81, 9.7) at (8.88, -8.89, 9.7) at (23.25, -10.16, 9.7) at (3.8, -26.67, 9.7) at (6.34, -1.27, 9.7) at (11.42, -6.35, 9.7) at (6.34, 6.35, 9.7) at (11.42, -8.89, 9.7) at (6.34, -21.59, 9.7) at (13.96, 1.27, 9.7) at (6.34, 26.67, 9.7) at (3.8, 3.81, 9.7) at (23.25, 12.7, 9.7) at (11.42, -31.75, 9.7) at (13.96, -19.05, 9.7) at (13.96, 26.67, 9.7) at (11.42, -13.97, 9.7) at (13.96, -24.13, 9.7) at (11.42, 13.97, 9.7) at (11.42, 11.43, 9.7) at (13.96, 24.13, 9.7) at (23.25, -15.24, 9.7) at (8.88, 6.35, 9.7) at (20.71, 12.7, 9.7) at (20.71, -20.32, 9.7) at (20.71, 33.02, 9.7) at (11.42, 34.29, 9.7) at (20.71, 10.16, 9.7) at (8.88, -13.97, 9.7) at (11.42, 19.05, 9.7) at (23.25, -30.48, 9.7) at (3.8, 29.21, 9.7) at (20.71, -12.7, 9.7) at (13.96, 34.29, 9.7) at (11.42, 31.75, 9.7) at (6.34, 31.75, 9.7) at (11.42, -34.29, 9.7) at (23.25, 20.32, 9.7) at (13.96, -36.83, 9.7) at (11.42, -11.43, 9.7) at (13.96, -26.67, 9.7) at (13.96, -31.75, 9.7) at (6.34, -29.21, 9.7) at (8.88, -6.35, 9.7) at (13.96, 16.51, 9.7) at (13.96, 36.83, 9.7) at (23.25, 30.48, 9.7) at (13.96, 19.05, 9.7) at (6.34, 3.81, 9.7) at (6.34, 19.05, 9.7) at (13.96, 31.75, 9.7) at (13.96, -6.35, 9.7) at (11.42, -29.21, 9.7) at (13.96, -13.97, 9.7) at (3.8, -21.59, 9.7) at (20.71, -27.94, 9.7) at (3.8, 36.83, 9.7) at (3.8, 24.13, 9.7) at (8.88, 36.83, 9.7) at (6.34, 36.83, 9.7) at (11.42, -24.13, 9.7) at (11.42, -36.83, 9.7) at (20.71, -15.24, 9.7) at (3.8, 31.75, 9.7) at (8.88, 21.59, 9.7) at (8.88, -36.83, 9.7) at (20.71, -35.56, 9.7) at (23.25, -25.4, 9.7) at (8.88, 24.13, 9.7) at (20.71, 27.94, 9.7) at (13.96, -34.29, 9.7) at (23.25, -35.56, 9.7) at (20.71, 30.48, 9.7) at (11.42, 26.67, 9.7) at (23.25, -20.32, 9.7) at (6.34, -24.13, 9.7) at (11.42, -16.51, 9.7) at (3.8, 8.89, 9.7) at (20.71, 25.4, 9.7) at (3.8, -11.43, 9.7) at (8.88, -11.43, 9.7) at (23.25, -33.02, 9.7) at (20.71, 2.54, 9.7) at (3.8, 6.35, 9.7) at (3.8, -36.83, 9.7) at (3.8, -6.35, 9.7) at (11.42, 3.81, 9.7) at (3.8, -24.13, 9.7) at (8.88, 13.97, 9.7) at (20.71, -2.54, 9.7) at (13.96, 11.43, 9.7) at (6.34, 11.43, 9.7) at (8.88, 34.29, 9.7) at (20.71, -30.48, 9.7) at (3.8, -3.81, 9.7) at (23.25, 33.02, 9.7) at (8.88, 19.05, 9.7) at (11.42, -19.05, 9.7) at (3.8, -34.29, 9.7) at (11.42, 21.59, 9.7) at (6.34, 24.13, 9.7) at (8.88, 29.21, 9.7) at (13.96, -16.51, 9.7) at (20.71, 0, 9.7) at (6.34, 21.59, 9.7) at (20.71, 35.56, 9.7) at (3.8, 21.59, 9.7) at (8.88, -21.59, 9.7) at (11.42, -21.59, 9.7) at (8.88, -24.13, 9.7) at (23.25, 15.24, 9.7) at (23.25, 5.08, 9.7) at (20.71, -25.4, 9.7) at (11.42, 36.83, 9.7) at (8.88, 8.89, 9.7) at (20.71, 20.32, 9.7) at (13.96, 3.81, 9.7) at (13.96, -29.21, 9.7) at (6.34, 29.21, 9.7) at (23.25, 35.56, 9.7) at (11.42, 16.51, 9.7) at (11.42, -3.81, 9.7) at (3.8, 34.29, 9.7) at (13.96, 29.21, 9.7) at (8.88, -16.51, 9.7) at (23.25, 27.94, 9.7) at (20.71, -17.78, 9.7) at (20.71, -5.08, 9.7) at (6.34, -31.75, 9.7) at (13.96, -8.89, 9.7) at (3.8, 11.43, 9.7) at (6.34, -19.05, 9.7) at (6.34, -3.81, 9.7) at (20.71, 5.08, 9.7) at (6.34, -36.83, 9.7) at (6.34, -13.97, 9.7) at (8.88, 1.27, 9.7) at (3.8, 13.97, 9.7) at (3.8, -1.27, 9.7) at (11.42, -1.27, 9.7) at (13.96, 13.97, 9.7) at (8.88, -19.05, 9.7) at (23.25, 10.16, 9.7) at (8.88, -3.81, 9.7) at (8.88, -34.29, 9.7) at (23.25, -2.54, 9.7) at (23.25, -12.7, 9.7) at (6.34, 1.27, 9.7) at (8.88, 16.51, 9.7) at (23.25, -5.08, 9.7) at (23.25, -27.94, 9.7) at (11.42, 24.13, 9.7) at (11.42, 29.21, 9.7) at (8.88, 31.75, 9.7) at (13.96, 8.89, 9.7) at (11.42, 8.89, 9.7) at (6.34, -8.89, 9.7) at (3.8, -31.75, 9.7) at (13.96, 21.59, 9.7) at (6.34, 16.51, 9.7) at (3.8, -13.97, 9.7) at (11.42, 6.35, 9.7) at (13.96, -11.43, 9.7) at (3.8, 19.05, 9.7) at (6.34, -34.29, 9.7) at (13.96, -1.27, 9.7) at (20.71, -10.16, 9.7) at (3.8, -19.05, 9.7) at (11.42, -26.67, 9.7) direction (0, 0, -1) diameter 1.524 depth 7 tip angle 180 bodies 1
chamfer "Chamfer1" distance 0.5 angle 45 8 edges at (26.4, 0, 9.7) (13.75, 40.65, 9.7) (1.1, 0, 9.7) (13.75, -40.65, 9.7) (-13.75, -40.65, 9.7) (-1.1, 0, 9.7) (-13.75, 40.65, 9.7) (-26.4, 0, 9.7) on bodies 1
extrude "Extrude4" add sketch "base" against normal blind 3.175 separate body makes body 2
extrude "Extrude5" add 1 faces at (-8.8, -40.65, -1.0583) along direction (0, -1, 0) blind 3.175 on bodies 2 bodies 2
extrude "Extrude6" add 1 faces at (8.8, 40.65, -1.0583) along direction (0, 1, 0) blind 3.175 on bodies 2 bodies 2
extrude "Extrude7" add 1 faces at (26.4, 14.6083, -1.0583) along direction (1, 0, 0) blind 3.175 on bodies 2 bodies 2
extrude "Extrude8" add 1 faces at (-26.4, 14.6083, -1.0583) along direction (-1, 0, 0) blind 3.175 on bodies 2 bodies 2
extrude "Extrude9" cut 1 faces at (-29.575, 14.6083, -1.0583) along direction (1, 0, 0) blind 3.175 on bodies 2 bodies 2
extrude "Extrude10" cut 1 faces at (10.9167, -43.825, -1.0583) along direction (0, 1, 0) blind 3.175 on bodies 2 bodies 2
extrude "Extrude11" add 1 faces at (-26.4, -12.4917, -1.0583) along direction (-1, 0, 0) blind 5.775 on bodies 2 bodies 2
extrude "Extrude12" add 1 faces at (-11.5917, -40.65, -2.1167) along direction (0, -1, 0) blind 5.775 on bodies 2 bodies 2
extrude "Extrude13" cut 1 faces at (-11.5917, -46.425, -2.1167) along direction (0, 1, 0) blind 1 on bodies 2 bodies 2
extrude "Extrude14" cut 1 faces at (-32.175, -15.675, -1.0583) along direction (1, 0, 0) blind 1 on bodies 2 bodies 2
sketch "bot wall" plane through (0, 0, 0) normal (0, 0, 1) x (1, 0, 0)
  line L0 (-31.175, 43.825) -> (-31.175, -45.425)
  line L1 (-31.175, -45.425) -> (29.575, -45.425)
  line L2 (29.575, -45.425) -> (29.575, 43.825)
  line L3 (29.575, 43.825) -> (-31.175, 43.825)
  line L4 (-31.175, -45.425) -> (29.575, -45.425)
  line L5 (29.575, -45.425) -> (29.575, -42.25)
  line L6 (29.575, -42.25) -> (-31.175, -42.25)
  line L7 (-31.175, -42.25) -> (-31.175, -45.425)
  line L8 (29.575, -42.25) -> (26.4, -42.25)
  line L9 (26.4, -42.25) -> (26.4, -45.425)
  line L10 (26.4, -45.425) -> (29.575, -45.425)
  line L11 (29.575, -45.425) -> (29.575, -42.25)
  line L12 (-31.175, -45.425) -> (-28, -45.425)
  line L13 (-28, -45.425) -> (-28, -42.25)
  line L14 (-28, -42.25) -> (-31.175, -42.25)
  line L15 (-31.175, -42.25) -> (-31.175, -45.425)
  dimension "d90" = 3.175
  dimension "d91" = 3.175
  dimension "d92" = 3.175
  dimension "d109" = 3.175
  constraint horizontal L4
  constraint vertical L5
  constraint horizontal L6
  constraint vertical L7
  constraint coincident L0.end L1.start
  constraint horizontal L8
  constraint vertical L9
  constraint horizontal L10
  constraint vertical L11
  constraint coincident L4 L9.end
  constraint horizontal L12
  constraint vertical L13
  constraint horizontal L14
  constraint vertical L15
  constraint coincident L6 L13.end
  measures "d90" distance of L4 L6
  measures "d91" distance of L1.end L5.end
  measures "d92" distance of L5.end L8.end
  measures "d109" distance of L7 L13
extrude "Extrude15" add sketch "bot wall" along normal blind 9.7 separate body contours L0 L1 L4 L6 L7 L12 L13 L14 L15 | L1 L4 L6 L9 L13 | L1 L2 L4 L5 L6 L8 L9 L10 L11 makes body 3
extrude "Extrude16" cut sketch "bot wall" along normal blind 3 contours L1 L2 L4 L5 L6 L8 L9 L10 L11 bodies 3
sketch "top of bot wall" plane through (0, 0, 9.7) normal (0, 0, 1) x (1, 0, 0)
  line L0 (-31.175, -42.25) -> (-31.175, -45.425)
  line L1 (-31.175, -45.425) -> (29.575, -45.425)
  line L2 (29.575, -45.425) -> (29.575, -42.25)
  line L3 (29.575, -42.25) -> (-31.175, -42.25)
  line L4 (29.575, -42.25) -> (26.4, -42.25)
  line L5 (26.4, -42.25) -> (26.4, -45.425)
  line L6 (26.4, -45.425) -> (29.575, -45.425)
  line L7 (29.575, -45.425) -> (29.575, -42.25)
  line L8 (-31.175, -45.425) -> (29.575, -45.425)
  line L9 (-31.175, -45.425) -> (-28, -45.425)
  line L10 (-28, -45.425) -> (-28, -42.25)
  line L11 (-28, -42.25) -> (-31.175, -42.25)
  line L12 (-31.175, -42.25) -> (-31.175, -45.425)
  dimension "d95" = 3.175
  dimension "d112" = 3.175
  constraint horizontal L4
  constraint vertical L5
  constraint horizontal L6
  constraint vertical L7
  constraint coincident L2.end L3.start
  constraint collinear L6 L8
  constraint horizontal L9
  constraint vertical L10
  constraint horizontal L11
  constraint vertical L12
  constraint coincident L3 L10.end
  constraint coincident L0.end L1.start
  measures "d95" distance of L2.end L4.end
  measures "d112" distance of L10 L12
extrude "Extrude17" cut sketch "top of bot wall" against normal blind 3 contours L1 L2 L3 L4 L5 L6 L7 L8 bodies 3
sketch "Sketch12" plane through (0, 0, 0) normal (0, 0, 1) x (1, 0, 0)
sketch "Sketch13" plane through (0, 0, 0) normal (0, 0, 1) x (1, 0, 0)
  line L0 (29.575, 43.825) -> (26.4, 43.825)
  line L1 (26.4, 43.825) -> (26.4, -45.425)
  line L2 (26.4, -45.425) -> (29.575, -45.425)
  line L3 (29.575, -45.425) -> (29.575, 43.825)
  line L4 (29.575, -45.425) -> (29.575, 43.825)
  line L5 (26.4, -42.25) -> (26.4, -45.425)
  line L6 (-31.175, -45.425) -> (29.575, -45.425)
  line L7 (29.575, 43.825) -> (-31.175, 43.825)
  constraint horizontal L0
  constraint vertical L1
  constraint horizontal L2
  constraint vertical L3
  constraint collinear L3 L4
  constraint collinear L1 L5
  constraint collinear L2 L6
  constraint collinear L0 L7
extrude "Extrude18" add sketch "Sketch13" along normal blind 25 separate body makes body 4
extrude "Extrude19" add 1 faces at (27.4583, -45.425, 8.3333) along direction (0, -1, 0) blind 3 on bodies 4 bodies 4
sketch "Sketch14" plane through (26.4, 0, 0) normal (-1, 0, 0) x (0, 0, 1)
  line L0 (0, 43.825) -> (0, -48.425)
  line L1 (0, -48.425) -> (25, -48.425)
  line L2 (25, -48.425) -> (25, 43.825)
  line L3 (25, 43.825) -> (0, 43.825)
  line L4 (0, -42.25) -> (9.7, -42.25)
  line L5 (9.7, -42.25) -> (9.7, -45.425)
  line L6 (9.7, -45.425) -> (0, -45.425)
  line L7 (0, -45.425) -> (0, -42.25)
  line L8 (0, -42.25) -> (0, -45.425)
  line L9 (6.7, -42.25) -> (3, -42.25)
  line L10 (3, -42.25) -> (3, -45.425)
  line L11 (3, -45.425) -> (6.7, -45.425)
  line L12 (6.7, -45.425) -> (6.7, -42.25)
  dimension "d102" = 3
  dimension "d103" = 3.175
  dimension "d104" = 9.7
  dimension "d105" = 3
  dimension "d106" = 3
  constraint horizontal L4
  constraint vertical L5
  constraint horizontal L6
  constraint vertical L7
  constraint coincident L0 L4.start
  constraint horizontal L9
  constraint vertical L10
  constraint horizontal L11
  constraint vertical L12
  constraint coincident L6 L10.end
  constraint coincident L4 L9.start
  measures "d102" distance of L0.end L6
  measures "d103" distance of L4 L6
  measures "d104" distance of L5 L8
  measures "d105" distance of L5 L12
  measures "d106" distance of L8 L10
extrude "Extrude20" cut sketch "Sketch14" against normal blind 3.175 contours L4 L6 L9 L10 L11 L12 bodies 4
extrude "Extrude21" cut sketch "bot wall" along normal blind 3 contours L0 L1 L4 L6 L7 L12 L13 L14 L15 bodies 3
extrude "Extrude22" cut sketch "top of bot wall" against normal blind 3 contours L0 L1 L3 L8 L9 L10 L11 L12 bodies 3
copy_body "CopyPasteBodies2" bodies 4 makes body 5
move_body "Move2" bodies 5 to x (1, 0, 0) y (0, 1, 0) z (0, 0, 1) at (-57.575, 0, 0)
extrude "Extrude23" add 1 faces at (28.5167, 43.825, 8.3333) along direction (0, 1, 0) blind 3 on bodies 4 bodies 4
extrude "Extrude24" add 1 faces at (-29.0583, 43.825, 8.3333) along direction (0, 1, 0) blind 3 on bodies 5 bodies 5
copy_body "CopyPasteBodies3" bodies 3 makes body 6
move_body "Move3" bodies 6 to x (1, 0, 0) y (0, 1, 0) z (0, 0, 1) at (0, 86.075, 0)
sketch "Sketch15" plane through (0, 0, 9.7) normal (0, 0, 1) x (1, 0, 0)
  line L0 (-28, 43.825) -> (-28, 40.65)
  line L1 (-28, 40.65) -> (26.4, 40.65)
  line L2 (26.4, 40.65) -> (26.4, 43.825)
  line L3 (26.4, 43.825) -> (-28, 43.825)
  line L4 (26.4, 43.825) -> (10, 43.825)
  line L5 (10, 43.825) -> (10, 40.65)
  line L6 (10, 40.65) -> (26.4, 40.65)
  line L7 (26.4, 40.65) -> (26.4, 43.825)
  dimension "d119" = 16.4
  dimension "d120" = 3.175
  constraint horizontal L4
  constraint vertical L5
  constraint horizontal L6
  constraint vertical L7
  constraint coincident L2.end L3.start
  measures "d119" distance of L2.end L4.end
  measures "d120" distance of L2.end L1.end
extrude "Extrude25" add sketch "Sketch15" along normal blind 15.3 separate body contours L1 L2 L3 L4 L5 L6 L7 makes body 7
copy_body "CopyPasteBodies4" bodies 7 makes body 8
move_body "Move4" bodies 8 to x (1, 0, 0) y (0, 1, 0) z (0, 0, 1) at (-36.4, 0, 0)
extrude "Extrude26" add 1 faces at (-26.4, 42.7667, 14.8) along direction (-1, 0, 0) blind 1.6 separate body on bodies 8 makes body 9
combine "Combine1" operation add target body 8 tool bodies 9
combine "Combine2" operation add target body 7 tool bodies 6
combine "Combine3" operation add target body 8 tool bodies 7
sketch "Sketch16" plane through (-28, 0, 0) normal (-1, 0, 0) x (0, 0, 1)
  line L0 (6.7, 40.65) -> (25, 40.65)
  line L1 (25, 40.65) -> (25, 43.825)
  line L2 (25, 43.825) -> (6.7, 43.825)
  line L3 (6.7, 43.825) -> (6.7, 40.65)
  line L4 (25, 40.65) -> (22, 40.65)
  line L5 (22, 40.65) -> (18.3, 40.65)
  line L6 (18.3, 40.65) -> (18.3, 43.825)
  line L7 (18.3, 43.825) -> (22, 43.825)
  line L8 (22, 43.825) -> (22, 40.65)
  dimension "d125" = 3
  dimension "d126" = 3.7
  dimension "d127" = 3.175
  constraint coincident L0.end L1.start
  constraint perpendicular L1 L4
  constraint horizontal L5
  constraint vertical L6
  constraint horizontal L7
  constraint vertical L8
  measures "d125" distance of L0.end L4.end
  measures "d126" distance of L4.end L5.end
  measures "d127" distance of L4.end L7.end
extrude "Extrude27" add sketch "Sketch16" along normal blind 3.175 contours L0 L2 L5 L6 L7 L8 bodies 8
sketch "Sketch17" plane through (26.4, 0, 0) normal (1, 0, 0) x (0, 0, -1)
  line L0 (-6.7, 43.825) -> (-25, 43.825)
  line L1 (-25, 43.825) -> (-25, 40.65)
  line L2 (-25, 40.65) -> (-6.7, 40.65)
  line L3 (-6.7, 40.65) -> (-6.7, 43.825)
  line L4 (-25, 40.65) -> (-22, 40.65)
  line L5 (-22, 40.65) -> (-18.3, 40.65)
  line L6 (-18.3, 40.65) -> (-18.3, 43.825)
  line L7 (-18.3, 43.825) -> (-22, 43.825)
  line L8 (-22, 43.825) -> (-22, 40.65)
  dimension "d130" = 3
  dimension "d131" = 3.7
  dimension "d132" = 3.175
  constraint coincident L1.end L2.start
  constraint perpendicular L1 L4
  constraint horizontal L5
  constraint vertical L6
  constraint horizontal L7
  constraint vertical L8
  measures "d130" distance of L1.end L4.end
  measures "d131" distance of L4.end L5.end
  measures "d132" distance of L4.end L7.end
extrude "Extrude28" add sketch "Sketch17" along normal blind 3.175 contours L0 L2 L5 L6 L7 L8 bodies 8
combine "Combine4" operation cut target body 4 tool bodies 8 keep tools
combine "Combine5" operation cut target body 5 tool bodies 8 keep tools
extrude "Extrude29" add 1 faces at (9.325, -45.425, -1.0583) along direction (0, -1, 0) blind 3 separate body on bodies 2 makes body 10
combine "Combine6" operation add target body 2 tool bodies 10
extrude "Extrude30" add 1 faces at (-10.925, 43.825, -1.0583) along direction (0, 1, 0) blind 3 separate body on bodies 2 makes body 11
combine "Combine7" operation add target body 2 tool bodies 11
sketch "Sketch18" plane through (0, 0, 0) normal (0, 0, -1) x (-1, 0, 0)
  line L0 (28, 46.825) -> (28, -48.425)
  line L1 (28, -48.425) -> (31.175, -48.425)
  line L2 (31.175, -48.425) -> (31.175, 46.825)
  line L3 (31.175, 46.825) -> (28, 46.825)
  line L4 (0, 0) -> (28, 0)
  line L5 (28, 0) -> (28, 15)
  line L6 (28, 15) -> (31.175, 15)
  line L7 (31.175, 15) -> (31.175, -15)
  line L8 (31.175, -15) -> (28, -15)
  line L9 (28, -15) -> (28, 15)
  dimension "d139" = 15
  dimension "d140" = 30
  constraint coincident L4.start origin
  constraint coincident L0 L4.end
  constraint perpendicular L0 L4
  constraint perpendicular L4 L5
  constraint horizontal L6
  constraint vertical L7
  constraint horizontal L8
  constraint vertical L9
  measures "d139" distance of L4.end L5.end
  measures "d140" distance of L5.end L8.end
extrude "Extrude31" add sketch "Sketch18" along normal blind 3.175 separate body contours L0 L2 L5 L6 L7 L8 L9 makes body 12
copy_body "CopyPasteBodies5" bodies 12 makes body 13
move_body "Move5" bodies 13 to x (1, 0, 0) y (0, 1, 0) z (0, 0, 1) at (57.575, 0, 0)
combine "Combine8" operation add target body 4 tool bodies 13
combine "Combine9" operation add target body 5 tool bodies 12
sketch "Sketch19" plane through (0, 0, 0) normal (0, 0, -1) x (-1, 0, 0)
  line L0 (28, 40.65) -> (28, 43.825)
  line L1 (28, 43.825) -> (-26.4, 43.825)
  line L2 (-26.4, 43.825) -> (-26.4, 40.65)
  line L3 (-26.4, 40.65) -> (28, 40.65)
  line L4 (-26.4, 40.65) -> (-10, 40.65)
  line L5 (-10, 40.65) -> (10, 40.65)
  line L6 (10, 40.65) -> (10, 43.825)
  line L7 (10, 43.825) -> (-10, 43.825)
  line L8 (-10, 43.825) -> (-10, 40.65)
  dimension "d143" = 16.4
  dimension "d144" = 20
  dimension "d145" = 3.175
  constraint coincident L2.end L3.start
  constraint perpendicular L2 L4
  constraint horizontal L5
  constraint vertical L6
  constraint horizontal L7
  constraint vertical L8
  measures "d143" distance of L2.end L4.end
  measures "d144" distance of L4.end L5.end
  measures "d145" distance of L4.end L7.end
extrude "Extrude32" add sketch "Sketch19" along normal blind 3.175 separate body contours L1 L3 L5 L6 L7 L8 makes body 14
copy_body "CopyPasteBodies6" bodies 14 makes body 15
move_body "Move6" bodies 15 to x (1, 0, 0) y (0, 1, 0) z (0, 0, 1) at (0, -86.075, 0)
combine "Combine10" operation add target body 8 tool bodies 14
combine "Combine11" operation add target body 3 tool bodies 15
extrude "Extrude33" add 1 faces at (29.575, 15.075, -2.1167) along direction (1, 0, 0) blind 3 separate body on bodies 2 makes body 16